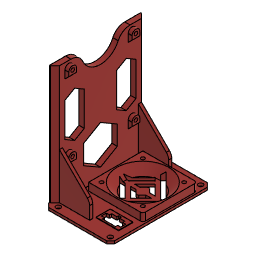
CPU Tray - RPi with Fan (Autodesk Fusion 360 design; units mm, degrees)
Autodesk Fusion 360 part; units mm, degrees
note: some values were not read from the file. Set by a fixed rule: which sketch regions a step uses.
sketch "Panel" plane through (92.9, 0, 0) normal (1, 0, 0) x (0, 1, 0)
  circle A0 centre (-9.085, 49.8044) radius 1.8
  circle A1 centre (-9.085, 9.5044) radius 1.8
  circle A2 centre (-79.085, 9.5044) radius 1.8
  circle A3 centre (-79.085, 49.8044) radius 1.8
  line L0 (-5.085, 6.0044) -> (-5.085, 51.0044)
  line L1 (-5.085, 51.0044) -> (-8.085, 54.0044)
  line L2 (-8.085, 54.0044) -> (-80.085, 54.0044)
  line L3 (-80.085, 54.0044) -> (-83.085, 51.0044)
  line L4 (-83.085, 51.0044) -> (-83.085, 6.0044)
  line L5 (-79.085, 49.8044) -> (-79.085, 9.5044) construction
  line L6 (-79.085, 9.5044) -> (-9.085, 9.5044) construction
  line L7 (-9.085, 9.5044) -> (-9.085, 49.8044) construction
  line L8 (-9.085, 49.8044) -> (-79.085, 49.8044) construction
  line L9 (-80.085, 3.0044) -> (-8.085, 3.0044)
  line L10 (-8.085, 3.0044) -> (-5.085, 6.0044)
  line L11 (-83.085, 6.0044) -> (-80.085, 3.0044)
  line L12 (-8.1678, 3.2044) -> (-5.285, 6.0872)
  line L13 (-5.285, 6.0872) -> (-5.285, 50.9215)
  line L14 (-5.285, 50.9215) -> (-8.1678, 53.8044)
  line L15 (-8.1678, 53.8044) -> (-80.0022, 53.8044)
  line L16 (-80.0022, 53.8044) -> (-82.885, 50.9215)
  line L17 (-82.885, 50.9215) -> (-82.885, 6.0872)
  line L18 (-82.885, 6.0872) -> (-80.0022, 3.2044)
  line L19 (-80.0022, 3.2044) -> (-8.1678, 3.2044) construction
  line L20 (-80.0022, 3.2044) -> (-79.8022, 3.0044)
  line L21 (-8.1678, 3.2044) -> (-8.3678, 3.0044) construction
  point P0 (-5.085, 3.0044)
  point P1 (-83.085, 3.0044)
  dimension "d5" = 78
  dimension "d10" = 70
  dimension "d11" = 40.3
  dimension "d14" = 3
  dimension "d15" = 3
  dimension "d16" = 3
  dimension "d17" = 3
  dimension "d18" = -0.2
  constraint coincident A3.centre L5.start
  constraint coincident A2.centre L5.end
  constraint coincident A1.centre L6.end
  constraint coincident A0.centre L7.end
  constraint perpendicular L0 L9
  constraint coincident P0 L9
  constraint coincident P0 L0
  constraint coincident P1 L4
  constraint coincident P1 L9
  constraint coincident L9 L20.end
  constraint parallel L18 L20
  constraint coincident L9 L21.end
  constraint parallel L12 L21
  measures "d5" distance of L0 L4
  measures "d10" distance of A3.centre A0.centre
  measures "d11" distance of A3.centre A2.centre
  measures "d14" distance of P0 L9.end
  measures "d15" distance of P0 L0.start
  measures "d16" distance of P1 L4.end
  measures "d17" distance of P1 L9.start
extrude "Extrude1" add sketch "Panel" along normal blind -1.5 and the other way blind -0.5
ref_plane "WorkPlane2" through (92.9, 0, 0) normal (1, 0, 0) x (0, 1, 0)
sketch "Tray" plane through (91.4, 0, 0) normal (-1, 0, 0) x (0, -1, 0)
  circle A0 centre (79.085, 9.5044) radius 1.8
  circle A1 centre (9.085, 9.5044) radius 1.8
  circle A2 centre (79.085, 49.8044) radius 1.8
  circle A3 centre (9.085, 49.8044) radius 1.8
  line L0 (80.085, 3.0044) -> (83.085, 6.0044)
  line L1 (83.085, 6.0044) -> (83.085, 51.0044)
  line L2 (83.085, 51.0044) -> (80.085, 54.0044)
  line L3 (80.085, 54.0044) -> (8.085, 54.0044)
  line L4 (8.085, 54.0044) -> (5.085, 51.0044)
  line L5 (5.085, 51.0044) -> (5.085, 6.0044)
  line L6 (5.085, 6.0044) -> (8.085, 3.0044)
  line L7 (8.085, 3.0044) -> (80.085, 3.0044)
  line L8 (79.335, 3.0044) -> (8.835, 3)
  line L9 (8.835, 3.7172) -> (8.835, 3)
  line L10 (8.835, 3.7172) -> (12.285, 7.1672)
  line L11 (12.285, 7.1672) -> (75.885, 7.1672)
  line L12 (44.085, 7.1672) -> (44.085, 3.0044) construction
  line L13 (79.335, 3.7172) -> (75.885, 7.1672)
  line L14 (79.335, 3.7172) -> (79.335, 3)
  dimension "d19" = 70.5
  dimension "d20" = 0.7171
  dimension "d21" = 4.879
  dimension "d22" = 63.6
  constraint perpendicular L6 L10
  constraint horizontal L11
  constraint midpoint L11 L12.start
  constraint midpoint L7 L12.end
  constraint symmetric L8.end L12 L14.end
  constraint symmetric L9.start L12 L13.start
  constraint symmetric L10.end L12 L11.end
  measures "d19" distance of L8.start L8.end
  measures "d20" distance of L8.end L9.start
  measures "d21" distance of L9.start L10.end
  measures "d22" distance of L10.end L11.end
extrude "Extrude2" add sketch "Tray" along normal blind 91.9 contours L7 L9 L10 L11 L13 L14
ref_plane "WorkPlane1" through (92.4, -75.885, 28.5044) normal (0, -1, 0) x (0, 0, 1)
sketch "Wall Brace" plane through (91.25, -75.885, 27.0044) normal (0, -1, 0) x (0, 0, 1)
  line L0 (27, -0.15) -> (-19.8372, -0.15)
  line L1 (-19.8372, 91.75) -> (-24, 91.75)
  line L2 (-24, -2.15) -> (27, -2.15)
  line L3 (1.8194, 13.9267) -> (-19.8392, 35.5853)
  line L4 (27, -0.15) -> (-39.2378, -0.15) construction
  line L5 (3.5768, 9.6869) -> (3.5814, -0.15)
  arc A0 (3.5768, 9.6869) -> (1.8194, 13.9267) centre (-2.4232, 9.6841) ccw
  line L6 (27, -2.15) -> (27, -0.15)
  line L7 (-19.8372, -0.15) -> (-19.8372, 91.75)
  line L8 (-24, 91.75) -> (-24, -2.15)
  dimension "d614" = 45
  dimension "d615" = 6
  constraint horizontal L4
  constraint coincident L0.start L4.start
  constraint midpoint L0 L5.end
  constraint tangent L3 A0
  constraint tangent L5 A0
  measures "d614" angle of L3 L4
  measures "d615" radius of A0
extrude "Extrude8" add sketch "Wall Brace" against normal blind 2.4 contours L0 L3 L5 A0 L7
extrude "Extrude9" add 1 faces at (74.796, -75.885, 14.3854) along direction (0, -1, 0) blind 2.4 from surface at -63.6
sketch "SPI Port" plane through (93.4, 0, 0) normal (1, 0, 0) x (0, 1, 0)
  circle A0 centre (-79.085, 9.5044) radius 1.8
  circle A1 centre (-9.085, 9.5044) radius 1.8
  circle A2 centre (-79.085, 49.8044) radius 1.8
  circle A3 centre (-9.085, 49.8044) radius 1.8
  line L0 (-83.085, 6.0044) -> (-80.085, 3.0044)
  line L1 (-80.085, 3.0044) -> (-8.085, 3.0044)
  line L2 (-8.085, 3.0044) -> (-5.085, 6.0044)
  line L3 (-5.085, 6.0044) -> (-5.085, 51.0044)
  line L4 (-5.085, 51.0044) -> (-8.085, 54.0044)
  line L5 (-8.085, 54.0044) -> (-80.085, 54.0044)
  line L6 (-80.085, 54.0044) -> (-83.085, 51.0044)
  line L7 (-83.085, 51.0044) -> (-83.085, 6.0044)
  line L8 (-53.25, 47.7) -> (-35.75, 47.7)
  line L9 (-35.75, 47.7) -> (-35.75, 36.7)
  line L10 (-35.75, 36.7) -> (-53.25, 36.7)
  line L11 (-53.25, 36.7) -> (-53.25, 47.7)
  line L12 (-39.4, 41.025) -> (-37, 41.025)
  line L13 (-37, 41.025) -> (-37, 44.775)
  line L14 (-39.4, 44.775) -> (-37, 44.775)
  line L15 (-39.4, 44.775) -> (-39.4, 46.475)
  line L16 (-39.4, 46.475) -> (-49.6, 46.475)
  line L17 (-49.6, 44.775) -> (-49.6, 46.475)
  line L18 (-52, 44.775) -> (-49.6, 44.775)
  line L19 (-52, 44.775) -> (-52, 41.025)
  line L20 (-49.6, 41.025) -> (-52, 41.025)
  line L21 (-49.6, 39.325) -> (-49.6, 41.025)
  line L22 (-45.5, 39.325) -> (-49.6, 39.325)
  line L23 (-45.5, 37.925) -> (-45.5, 39.325)
  line L24 (-43.5, 37.925) -> (-45.5, 37.925)
  line L25 (-43.5, 39.325) -> (-43.5, 37.925)
  line L26 (-39.4, 39.325) -> (-39.4, 41.025)
  line L27 (-43.5, 39.325) -> (-39.4, 39.325)
  line L28 (-49.6, 39.325) -> (-39.4, 39.325) construction
  line L29 (-44.5, 37.925) -> (-44.5, 46.475) construction
  line L30 (-52, 42.9) -> (-37, 42.9) construction
  line L31 (-49.6, 46.475) -> (-49.6, 39.325) construction
  line L32 (-39.4, 39.325) -> (-39.4, 46.475) construction
  line L33 (-37, 41.025) -> (-52, 41.025) construction
  line L34 (-52, 44.775) -> (-37, 44.775) construction
  dimension "d24" = 2
  dimension "d25" = 15
  dimension "d26" = 10.2
  constraint midpoint L24 L29.start
  constraint midpoint L16 L29.end
  constraint perpendicular L16 L29
  constraint symmetric L23 L25 L29
  constraint symmetric L21 L26 L29
  constraint symmetric L15 L17 L29
  constraint symmetric L13 L19 L29
  constraint symmetric L9 L11 L29
  constraint midpoint L19 L30.start
  constraint midpoint L13 L30.end
  constraint perpendicular L28 L31
  constraint perpendicular L16 L32
  constraint perpendicular L19 L33
  constraint perpendicular L19 L34
  constraint horizontal L34
  constraint vertical L31
  constraint vertical L32
  constraint vertical L26
  constraint vertical L17
  constraint horizontal L24
  constraint vertical L25
  measures "d24" distance of L23 L25
  measures "d25" distance of L13 L19
  measures "d26" distance of L21 L26
move_body "Move1" bodies 1 to x (0, 0, -1) y (0, 1, 0) z (1, 0, 0) at (90.3956, 0, 96.4044)
sketch "Screw Holes" plane through (97.5628, 0, 0) normal (1, 0, 0) x (0, 1, 0)
  line L0 (-14.685, 40.7377) -> (-12.285, 40.7377)
  line L1 (-12.285, 40.7377) -> (-12.285, 96.9044)
  line L2 (-12.285, 96.9044) -> (-75.885, 96.9044)
  line L3 (-75.885, 96.9044) -> (-75.885, 40.7377)
  line L4 (-75.885, 40.7377) -> (-73.485, 40.7377)
  line L5 (-73.485, 40.7377) -> (-73.485, 5.0044)
  line L6 (-73.485, 5.0044) -> (-14.685, 5.0044)
  line L7 (-14.685, 5.0044) -> (-14.685, 40.7377)
  line L8 (-44.085, 96.9044) -> (-44.085, 62.9044) construction
  line L9 (-19.585, 33.9044) -> (-68.585, 33.9044) construction
  line L10 (-68.585, 33.9044) -> (-68.585, 91.9044) construction
  line L11 (-68.585, 91.9044) -> (-19.585, 91.9044) construction
  line L12 (-19.585, 91.9044) -> (-19.585, 33.9044) construction
  line L13 (-19.585, 33.9044) -> (-68.585, 91.9044) construction
  line L14 (-68.585, 33.9044) -> (-19.585, 91.9044) construction
  circle A0 centre (-68.585, 91.9044) radius 1.4
  circle A1 centre (-19.585, 91.9044) radius 1.4
  circle A2 centre (-68.585, 33.9044) radius 1.4
  circle A3 centre (-19.585, 33.9044) radius 1.4
  line L15 (-65.585, 30.9044) -> (-71.585, 30.9044)
  line L16 (-71.585, 30.9044) -> (-71.585, 33.9044)
  line L17 (-65.585, 33.9044) -> (-65.585, 30.9044)
  line L18 (-71.585, 91.9044) -> (-71.585, 88.9044)
  line L19 (-71.585, 88.9044) -> (-65.585, 88.9044)
  line L20 (-65.585, 88.9044) -> (-65.585, 91.9044)
  arc A4 (-65.585, 91.9044) -> (-71.585, 91.9044) centre (-68.585, 91.9044) ccw
  arc A5 (-65.585, 33.9044) -> (-71.585, 33.9044) centre (-68.585, 33.9044) ccw
  line L21 (-16.585, 30.9044) -> (-16.585, 33.9044)
  arc A6 (-16.585, 33.9044) -> (-22.585, 33.9044) centre (-19.585, 33.9044) ccw
  line L22 (-22.585, 33.9044) -> (-22.585, 30.9044)
  line L23 (-22.585, 30.9044) -> (-16.585, 30.9044)
  line L24 (-16.585, 91.9044) -> (-16.585, 88.9044)
  line L25 (-16.585, 88.9044) -> (-22.585, 88.9044)
  arc A7 (-16.585, 91.9044) -> (-22.585, 91.9044) centre (-19.585, 91.9044) ccw
  line L26 (-22.585, 88.9044) -> (-22.585, 91.9044)
  point P0 (-68.585, 33.9044)
  dimension "d28" = 49
  dimension "d29" = 58
  dimension "d30" = 5
  dimension "d31" = 2.8
  dimension "d33" = 2.8
  dimension "d35" = 2.8
  dimension "d36" = 2.8
  dimension "d45" = 3
  dimension "d46" = 6
  dimension "d47" = 3
  dimension "d48" = 6
  dimension "d49" = 3
  dimension "d50" = 3
  constraint midpoint L2 L8.start
  constraint perpendicular L6 L8
  constraint horizontal L9
  constraint perpendicular L9 L10
  constraint parallel L9 L11
  constraint parallel L10 L12
  constraint coincident L13 L8.end
  constraint coincident L14 L8.end
  constraint coincident L10.end L11.start
  constraint coincident L11.end L12.start
  constraint coincident P0 L9.end
  constraint coincident L9.start L12.end
  constraint horizontal L15
  constraint perpendicular L15 L16
  constraint parallel L16 L17
  constraint coincident L9 L17.start
  constraint perpendicular L11 L18
  constraint perpendicular L18 L19
  constraint coincident L11 L20.end
  constraint tangent L20 A4
  constraint concentric A0 A4
  constraint concentric A2 A5
  constraint symmetric L8 L15.start L22.end
  constraint symmetric L8 L15.end L21.start
  constraint symmetric L8 L16.end L21.end
  constraint symmetric L8 L17.start A6.end
  constraint symmetric L8 L18.start L24.start
  constraint symmetric L8 L18.end L24.end
  constraint symmetric L8 L19.end L25.end
  constraint symmetric L8 L20.end A7.end
  constraint symmetric L8 A4 A7
  constraint symmetric L8 A5 A6
  measures "d28" distance of L10.end L11.end
  measures "d29" distance of P0 L10.end
  measures "d30" distance of L2 L11
  measures "d31" diameter of A0
  measures "d33" diameter of A1
  measures "d35" diameter of A2
  measures "d36" diameter of A3
  measures "d45" distance of L10.end L19
  measures "d46" distance of L18.end L19.end
  measures "d47" distance of L15.end L16.end
  measures "d48" distance of L15.start L15.end
  measures "d49" radius of A5
  measures "d50" radius of A4
extrude "Extrude10" cut sketch "Screw Holes" against normal blind 4.163 contours A0 | A1 | A2 | A3
extrude "Extrude11" add sketch "Screw Holes" along normal blind 3 contours L15 L16 L17 A5 | L18 L19 L20 A4 | L21 A6 L22 L23 | L24 L25 A7 L26
draft "Draft2" angle 45 neutral plane through (100.5628, 0, 0) pull (1, 0, 0) 4 faces at (98.5628, -69.585, 88.9044) (99.5628, -18.585, 88.9044) (98.5628, -67.585, 30.9044) (98.5628, -20.585, 30.9044)
sketch "Vertical Cutouts" plane through (97.5628, 0, 0) normal (1, 0, 0) x (0, 1, 0)
  line L0 (-16.585, 91.9044) -> (-16.585, 85.9044)
  line L1 (-16.585, 85.9044) -> (-22.585, 85.9044)
  line L2 (-22.585, 85.9044) -> (-22.585, 91.9044)
  arc A0 (-16.585, 91.9044) -> (-22.585, 91.9044) centre (-19.585, 91.9044) ccw
  line L3 (-65.585, 91.9044) -> (-65.585, 85.9044)
  line L4 (-65.585, 85.9044) -> (-71.585, 85.9044)
  line L5 (-71.585, 85.9044) -> (-71.585, 91.9044)
  arc A1 (-65.585, 91.9044) -> (-71.585, 91.9044) centre (-68.585, 91.9044) ccw
  line L6 (-22.585, 27.9044) -> (-22.585, 33.9044)
  arc A2 (-16.585, 33.9044) -> (-22.585, 33.9044) centre (-19.585, 33.9044) ccw
  line L7 (-16.585, 33.9044) -> (-16.585, 27.9044)
  line L8 (-16.585, 27.9044) -> (-22.585, 27.9044)
  line L9 (-65.585, 27.9044) -> (-71.585, 27.9044)
  line L10 (-71.585, 27.9044) -> (-71.585, 33.9044)
  arc A3 (-65.585, 33.9044) -> (-71.585, 33.9044) centre (-68.585, 33.9044) ccw
  line L11 (-65.585, 33.9044) -> (-65.585, 27.9044)
  line L12 (-14.685, 40.7377) -> (-12.285, 40.7377)
  line L13 (-12.285, 40.7377) -> (-12.285, 96.9044)
  line L14 (-12.285, 96.9044) -> (-75.885, 96.9044)
  line L15 (-75.885, 96.9044) -> (-75.885, 40.7377)
  line L16 (-75.885, 40.7377) -> (-73.485, 40.7377)
  line L17 (-73.485, 40.7377) -> (-73.485, 5.0044)
  line L18 (-73.485, 5.0044) -> (-14.685, 5.0044)
  line L19 (-14.685, 5.0044) -> (-14.685, 40.7377)
  line L20 (-44.085, 96.9044) -> (-44.085, 5.0044) construction
  line L21 (-56.585, 71.6243) -> (-64.085, 75.9544)
  line L22 (-64.085, 75.9544) -> (-71.585, 71.6243)
  line L23 (-71.585, 71.6243) -> (-71.585, 45.2845)
  line L24 (-71.585, 45.2845) -> (-64.085, 40.9544)
  line L25 (-64.085, 40.9544) -> (-56.585, 45.2845)
  line L26 (-56.585, 45.2845) -> (-56.585, 71.6243)
  line L27 (-64.085, 75.9544) -> (-64.085, 40.9544) construction
  line L28 (-24.085, 75.9544) -> (-16.585, 71.6243)
  line L29 (-16.585, 71.6243) -> (-16.585, 45.2845)
  line L30 (-16.585, 45.2845) -> (-24.085, 40.9544)
  line L31 (-24.085, 40.9544) -> (-31.585, 45.2845)
  line L32 (-31.585, 45.2845) -> (-31.585, 71.6243)
  line L33 (-31.585, 71.6243) -> (-24.085, 75.9544)
  line L34 (-73.485, 40.7377) -> (-73.485, 96.9044)
  line L35 (-14.685, 40.7377) -> (-14.685, 96.9044)
  line L36 (-44.085, 50.9544) -> (-44.085, 5.0044) construction
  line L37 (-44.085, 42.9794) -> (-57.0754, 35.4794)
  line L38 (-57.0754, 35.4794) -> (-57.0754, 20.4794)
  line L39 (-57.0754, 20.4794) -> (-44.085, 12.9794)
  line L40 (-44.085, 12.9794) -> (-31.0946, 20.4794)
  line L41 (-31.0946, 20.4794) -> (-31.0946, 35.4794)
  line L42 (-31.0946, 35.4794) -> (-44.085, 42.9794)
  line L43 (-44.085, 104.4044) -> (-44.085, 74.4044) construction
  line L44 (-31.0946, 96.9044) -> (-57.0754, 96.9044) construction
  circle A4 centre (-44.085, 96.9044) radius 15
  point P0 (-44.085, 50.9544)
  point P1 (-44.085, 27.9794)
  dimension "d56" = 15
  dimension "d57" = 15
  constraint midpoint L14 L20.start
  constraint midpoint L18 L20.end
  constraint midpoint L20 P0
  constraint symmetric L24 L25 L27
  constraint symmetric L21 L22 L27
  constraint symmetric L20 L22.end L28.end
  constraint symmetric L20 L21.end L28.start
  constraint symmetric L20 L24.end L30.end
  constraint symmetric L20 L25.end L31.end
  constraint symmetric L20 L23.end L29.end
  constraint symmetric L20 L21.start L32.end
  constraint coincident L16.end L17.start
  constraint coincident L14 L34.end
  constraint perpendicular L14 L34
  constraint coincident L12.start L19.end
  constraint coincident L14 L35.end
  constraint perpendicular L14 L35
  constraint coincident P0 L36.start
  constraint midpoint L36 P1
  constraint parallel L20 L43
  constraint collinear L14 L44
  constraint coincident L20.start A4.centre
  measures "d56" distance of L23 L26
  measures "d57" distance of L37.start P1
extrude "Extrude12" cut sketch "Vertical Cutouts" against normal blind 4.163 contours L14 A4 | L21 L22 L23 L24 L25 L26 | L28 L29 L30 L31 L32 L33 | L37 L38 L39 L40 L41 L42 picked at (-39.9538, 94.0878)
fillet "Fillet4" radius 10 2 edges at (95.4814, -59.085, 96.9044) (95.4814, -29.085, 96.9044)
sketch "Fan and SPI Sport" plane through (0, 0, 5.0044) normal (0, 0, 1) x (-1, 0, 0)
  line L0 (-120.9814, 14.685) -> (-97.5628, 14.685)
  line L1 (-97.5628, 14.685) -> (-97.5628, 73.485)
  line L2 (-97.5628, 73.485) -> (-120.9814, 73.485)
  line L3 (-120.9814, 73.485) -> (-120.9814, 75.885)
  line L4 (-120.9814, 75.885) -> (-97.5628, 75.885)
  line L5 (-97.5628, 75.885) -> (-94.1128, 79.335)
  line L6 (-94.1128, 79.335) -> (-93.4, 79.335)
  line L7 (-93.4, 79.335) -> (-93.4, 80.085)
  line L8 (-93.4, 80.085) -> (-96.4, 83.085)
  line L9 (-96.4, 83.085) -> (-141.4, 83.085)
  line L10 (-141.4, 83.085) -> (-144.4, 80.085)
  line L11 (-144.4, 80.085) -> (-144.4, 8.085)
  line L12 (-144.4, 8.085) -> (-141.4, 5.085)
  line L13 (-141.4, 5.085) -> (-96.4, 5.085)
  line L14 (-96.4, 5.085) -> (-93.4, 8.085)
  line L15 (-93.4, 8.085) -> (-93.4, 8.835)
  line L16 (-93.4, 8.835) -> (-94.1128, 8.835)
  line L17 (-94.1128, 8.835) -> (-97.5628, 12.285)
  line L18 (-97.5628, 12.285) -> (-120.9814, 12.285)
  line L19 (-120.9814, 12.285) -> (-120.9814, 14.685)
  circle A0 centre (-99.9, 79.085) radius 1.8
  circle A1 centre (-140.2, 79.085) radius 1.8
  circle A2 centre (-99.9, 9.085) radius 1.8
  circle A3 centre (-140.2, 9.085) radius 1.8
  line L20 (-101.0628, 56.735) -> (-143.0628, 56.735)
  line L21 (-143.0628, 56.735) -> (-143.0628, 14.735)
  line L22 (-143.0628, 14.735) -> (-101.0628, 14.735)
  line L23 (-122.0628, 56.735) -> (-122.0628, 14.735) construction
  circle A4 centre (-122.0628, 35.735) radius 20
  line L24 (-106.0628, 19.735) -> (-138.0628, 19.735) construction
  line L25 (-138.0628, 19.735) -> (-138.0628, 51.735) construction
  line L26 (-138.0628, 51.735) -> (-106.0628, 51.735) construction
  line L27 (-106.0628, 51.735) -> (-106.0628, 19.735) construction
  line L28 (-106.0628, 19.735) -> (-138.0628, 51.735) construction
  line L29 (-138.0628, 19.735) -> (-106.0628, 51.735) construction
  circle A5 centre (-138.0628, 19.735) radius 1.4
  circle A6 centre (-106.0628, 19.735) radius 1.4
  circle A7 centre (-106.0628, 51.735) radius 1.4
  circle A8 centre (-138.0628, 51.735) radius 1.4
  line L30 (-121.75, 60.7) -> (-139.25, 60.7)
  line L31 (-139.25, 60.7) -> (-139.25, 71.7)
  line L32 (-139.25, 71.7) -> (-121.75, 71.7)
  line L33 (-121.75, 71.7) -> (-121.75, 60.7)
  line L34 (-135.6, 70.475) -> (-135.6, 63.325) construction
  line L35 (-125.4, 63.325) -> (-125.4, 70.475) construction
  line L36 (-135.6, 63.325) -> (-125.4, 63.325) construction
  line L37 (-135.6, 65.025) -> (-138, 65.025)
  line L38 (-135.6, 63.325) -> (-135.6, 65.025)
  line L39 (-131.5, 63.325) -> (-135.6, 63.325)
  line L40 (-131.5, 61.925) -> (-131.5, 63.325)
  line L41 (-129.5, 61.925) -> (-131.5, 61.925)
  line L42 (-129.5, 63.325) -> (-129.5, 61.925)
  line L43 (-129.5, 63.325) -> (-125.4, 63.325)
  line L44 (-125.4, 63.325) -> (-125.4, 65.025)
  line L45 (-125.4, 65.025) -> (-123, 65.025)
  line L46 (-123, 65.025) -> (-123, 68.775)
  line L47 (-125.4, 68.775) -> (-123, 68.775)
  line L48 (-125.4, 68.775) -> (-125.4, 70.475)
  line L49 (-125.4, 70.475) -> (-135.6, 70.475)
  line L50 (-135.6, 68.775) -> (-135.6, 70.475)
  line L51 (-138, 68.775) -> (-135.6, 68.775)
  line L52 (-138, 68.775) -> (-138, 65.025)
  line L53 (-101.0628, 56.735) -> (-101.0628, 14.735)
  point P0 (-122.0628, 35.735)
  dimension "d65" = 40
  dimension "d66" = 32
  dimension "d67" = 32
  dimension "d68" = 2.8
  dimension "d69" = 2.8
  dimension "d70" = 2.8
  dimension "d71" = 2.8
  dimension "d72" = 2
  dimension "d73" = 15
  dimension "d74" = 10.2
  dimension "d93" = 42
  constraint horizontal L20
  constraint vertical L21
  constraint horizontal L22
  constraint midpoint L22 L23.end
  constraint midpoint L23 P0
  constraint horizontal L24
  constraint perpendicular L24 L25
  constraint parallel L24 L26
  constraint parallel L25 L27
  constraint coincident L28 P0
  constraint coincident L29 P0
  constraint coincident P0 A4.centre
  constraint coincident L24.end L25.start
  constraint coincident L24.start L27.end
  constraint coincident L26.end L27.start
  constraint coincident L25.end L26.start
  constraint perpendicular L34 L36
  constraint perpendicular L35 L49
  constraint vertical L23
  constraint midpoint L20 L23.start
  measures "d65" diameter of A4
  measures "d66" distance of L25.end L26.end
  measures "d67" distance of L24.end L25.end
  measures "d68" diameter of A5
  measures "d69" diameter of A6
  measures "d70" diameter of A8
  measures "d71" diameter of A7
  measures "d72" distance of L40 L42
  measures "d73" distance of L46 L52
  measures "d74" distance of L38 L44
  measures "d93" distance of L20.end L20.start
extrude "Extrude13" add sketch "Fan and SPI Sport" along normal blind 6 contours L20 L21 L22 L53
draft "Draft3" angle 45 neutral plane through (0, 0, 11.0044) pull (0, 0, 1) 1 faces at (102.1622, -33.7436, 7.0044)
sketch "Fan Grill" plane through (0, 0, 3.0044) normal (0, 0, -1) x (1, 0, 0)
  circle A0 centre (99.9, 79.085) radius 1.8
  circle A1 centre (140.2, 79.085) radius 1.8
  circle A2 centre (99.9, 9.085) radius 1.8
  circle A3 centre (140.2, 9.085) radius 1.8
  line L0 (96.4, 83.085) -> (93.4, 80.085)
  line L1 (93.4, 80.085) -> (93.4, 8.085)
  line L2 (93.4, 8.085) -> (96.4, 5.085)
  line L3 (96.4, 5.085) -> (141.4, 5.085)
  line L4 (141.4, 5.085) -> (144.4, 8.085)
  line L5 (144.4, 8.085) -> (144.4, 80.085)
  line L6 (144.4, 80.085) -> (141.4, 83.085)
  line L7 (141.4, 83.085) -> (96.4, 83.085)
  circle A4 centre (122.0628, 35.735) radius 14
  line L8 (134.3201, 34.235) -> (119.9415, 19.8563)
  line L9 (140.0628, 35.735) -> (104.0628, 35.735) construction
  line L10 (109.8054, 37.235) -> (105.5628, 37.235)
  line L11 (125.8349, 34.235) -> (130.0775, 34.235)
  line L12 (109.8054, 34.235) -> (105.5628, 34.235)
  line L13 (118.2907, 37.235) -> (114.0481, 37.235)
  line L14 (130.0775, 34.235) -> (122.0628, 26.2203)
  line L15 (125.8349, 34.235) -> (123.1234, 31.5236)
  arc A5 (121.0021, 31.5236) -> (123.1234, 31.5236) centre (122.0628, 32.5842) ccw
  line L16 (104.0628, 35.735) -> (122.0628, 17.735)
  line L17 (134.3201, 34.235) -> (138.5628, 34.235)
  line L18 (130.0775, 37.235) -> (122.0628, 45.2497)
  line L19 (140.0628, 35.735) -> (122.0628, 17.735)
  line L20 (134.3201, 37.235) -> (119.9415, 51.6137)
  arc A6 (123.1234, 39.9464) -> (121.0021, 39.9464) centre (122.0628, 38.8858) ccw
  line L21 (125.8349, 37.235) -> (123.1234, 39.9464)
  line L22 (118.2907, 34.235) -> (121.0021, 31.5236)
  line L23 (140.0628, 35.735) -> (122.0628, 53.735)
  line L24 (118.2907, 34.235) -> (114.0481, 34.235)
  line L25 (125.8349, 37.235) -> (130.0775, 37.235)
  line L26 (114.0481, 34.235) -> (122.0628, 26.2203)
  line L27 (122.0628, 53.735) -> (122.0628, 17.735) construction
  line L28 (119.9415, 47.371) -> (117.8201, 49.4924)
  line L29 (119.9415, 24.099) -> (117.8201, 21.9776)
  line L30 (114.0481, 37.235) -> (122.0628, 45.2497)
  line L31 (118.2907, 37.235) -> (121.0021, 39.9464)
  line L32 (104.0628, 35.735) -> (122.0628, 53.735)
  line L33 (109.8054, 37.235) -> (119.9415, 47.371)
  line L34 (109.8054, 34.235) -> (119.9415, 24.099)
  line L35 (134.3201, 37.235) -> (138.5628, 37.235)
  point P0 (138.5628, 40.235)
  point P1 (122.0628, 30.4629)
  point P2 (122.0628, 35.735)
  dimension "d83" = 3
  dimension "d2" = 3
  dimension "d3" = 36
  dimension "d4" = 36
  dimension "d87" = 5.3345
  dimension "d6" = 1.5
  constraint coincident L35.end L23
  constraint coincident L17.end L19
  constraint coincident L19.end L16
  constraint coincident L9.end L16
  constraint coincident L9.end L32
  constraint coincident L27.start L23
  constraint coincident L23.end L32
  constraint coincident L9.start L23
  constraint coincident L9.start L19
  constraint coincident L16.end L19
  constraint parallel L8 L19
  constraint coincident L8.end L16
  constraint symmetric L9 L16 L32
  constraint symmetric L9 L19 L23
  constraint symmetric L9 L17 L35
  constraint midpoint P2 L9
  constraint symmetric L8.end L20.end L9
  constraint symmetric L20.start L8.start L9
  constraint perpendicular L14 L26
  constraint perpendicular L15 L22
  constraint coincident L14.end L26
  constraint coincident L26.end L14
  constraint coincident P1 L22
  constraint coincident L22.start L24
  constraint coincident L24.start L22
  constraint coincident L24.end L26
  constraint coincident L26.start L24
  constraint coincident L15.start L11
  constraint coincident L11.start L15
  constraint coincident L14.start L11
  constraint coincident L11.end L14
  constraint collinear L11 L24
  constraint symmetric L14 L26 L27
  constraint symmetric L15 L22 L27
  constraint coincident P1 L15
  constraint tangent L15 A5
  constraint tangent A5 L22
  constraint symmetric L13.end L24.end L9
  constraint symmetric L18.end L14.end L9
  constraint symmetric L13.start L22.start L9
  constraint symmetric L21.start L11.start L9
  constraint symmetric L11.start L21.start L9
  constraint symmetric L11.end L18.start L9
  constraint symmetric A6.start L15.end L9
  constraint symmetric A6.end A5.start L9
  constraint symmetric L9 A5 A6
  constraint coincident L29.end L16
  constraint coincident L34.end L29
  constraint coincident L29.start L34
  constraint coincident L34.start L12
  constraint coincident L12.start L34
  constraint coincident L12.end L16
  constraint symmetric L10.start L12.start L9
  constraint symmetric L10.end L12.end L9
  constraint symmetric L29.start L28.start L9
  constraint symmetric L29.end L28.end L9
  constraint symmetric L28.start L29.start L9
  constraint coincident P2 L27
  measures "d83" distance of L8 L19
  measures "d2" distance of L17 L35
  measures "d3" distance of L16.end L23.end
  measures "d4" distance of L9.end L9.start
  measures "d87" distance of P1 L11.start
  measures "d6" radius of A5
extrude "Extrude16" cut sketch "Fan Grill" against normal blind 12 contours A4 L20 L23 L35 | A4 L23 L35 | A4 L17 L19 | A4 L8 L17 L19 | A4 L20 L23 L32 | A4 L8 L16 L19 | A4 L10 L28 L32 L33 | A4 L28 L32 | A4 L16 L29 | A4 L12 L16 L29 L34 | A4 L10 L32 | A4 L12 L16 | L11 L14 L15 A5 L22 L24 L26 | L13 L18 A6 L21 L25 L30 L31
fillet "Fillet5" radius 2 2 edges at (143.0628, -14.735, 8.0044) (143.0628, -56.735, 8.0044)
extrude "Extrude14" add sketch "Fan and SPI Sport" along normal blind 0.4 contours L30 L31 L32 L33
extrude "Extrude15" cut sketch "Fan and SPI Sport" against normal blind 2 contours L37 L38 L39 L40 L41 L42 L43 L44 L45 L46 L47 L48 L49 L50 L51 L52
equation "d15 = d14"
equation "d17 = d16"
equation "d33 = d31"
equation "d35 = d31"
equation "d69 = d68"
equation "d70 = d68"
equation "d71 = d68"
